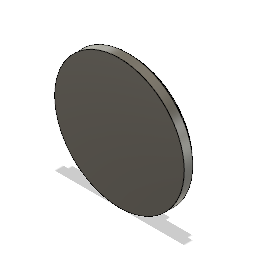
blackwidow v1 (Autodesk Fusion 360 design; units mm, degrees)
Autodesk Fusion 360 part; units mm, degrees
sketch "Sketch1" plane through (0, 0, 0) normal (0, 0, 1) x (1, 0, 0)
  circle A0 centre (0, 0) radius 75
  constraint coincident A0.centre origin
extrude "Extrude1" add sketch "Sketch1" along normal blind 10
sketch "Sketch2" plane through (0, 0, 0) normal (0, 0, 1) x (1, 0, 0)
  circle A0 centre (0, 0) radius 69.6419
  circle A1 centre (0, 0) radius 63.2456
  constraint coincident A0.centre A1.centre
  constraint concentric A0 A1
extrude "Extrude2" add sketch "Sketch2" against normal blind 5
sketch "Sketch3" plane through (0, 0, 0) normal (0, 0, 1) x (1, 0, 0)
  line L0 (-40, 50) -> (-35, 50)
  line L1 (-40, 50) -> (-37.5, 50)
  line L2 (40, 50) -> (-40, 50)
  line L3 (-37.5, 50) -> (-10, 0)
  line L4 (-10, 0) -> (-40, -50)
  line L5 (-40, -50) -> (40, -50)
  line L6 (40, -50) -> (10, 0)
  line L7 (40, 55) -> (10, 0)
  constraint midpoint L0 L1.end
  constraint parallel L0 L1
  constraint parallel L1 L2
  constraint parallel L2 L5
extrude "Extrude3" add 1 faces at (67.2505, -3.4599, -5) along direction (0, 0, 1) blind 5
extrude "Extrude4" add sketch "Sketch3" against normal blind 10
sketch "Sketch4" plane through (0, 0, 0) normal (0, 0, 1) x (1, 0, 0)
